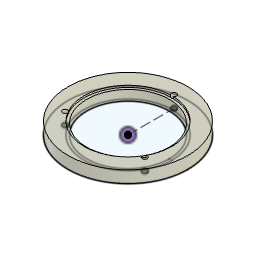
Kattolampun adapteri v5 (Autodesk Fusion 360 design; units mm, degrees)
Autodesk Fusion 360 part; units mm, degrees
sketch "Base" plane through (0, 0, 0) normal (0, 0, 1) x (1, 0, 0)
  circle A0 centre (0, 0) radius 45
  circle A1 centre (0, 0) radius 47.75
  circle A2 centre (0, 0) radius 65
  line L0 (0, 0) -> (0, 50) construction
  circle A3 centre (0, 50) radius 2.75
  circle A4 centre (-43.3013, -25) radius 2.75
  circle A5 centre (43.3013, -25) radius 2.75
  dimension "d6" = 90
  dimension "d7" = 95.5
  dimension "d8" = 130
  dimension "d12" = 50
  dimension "d13" = 5.5
  dimension "d15" = 360
  constraint coincident A0.centre A1.centre
  constraint vertical L0
  constraint coincident L0.end A3.centre
  measures "d6" diameter of A0
  measures "d7" diameter of A1
  measures "d8" diameter of A2
  measures "d12" distance of A0.centre L0.end
  measures "d13" diameter of A3
extrude "Extrude1" add sketch "Base" along normal blind 13 contours A0 | A1 A3 A4 A5 | A2
extrude "Extrude2" add sketch "Base" along normal up to surface (11 mm away) from surface at 2 contours A1 A3 A4 A5 | A1 A3 | A1 A5 | A1 A4 picked at (0, 47.5815) picked at (41.2068, -23.7907) picked at (-41.224, -23.7621)
extrude "Extrude3" add sketch "Base" along normal up to surface (5 mm away) from surface at 8 contours A1 A3 | A1 A3 | A1 A5 | A1 A5 | A1 A4 | A1 A4
extrude "Extrude4" cut sketch "Base" along normal up to surface (13 mm away) contours A1 A3 | A1 A5 | A1 A4 picked at (-0.0423, 49.4138) picked at (42.7651, -24.7549) picked at (-42.7945, -24.7074)
extrude "Extrude5" cut sketch "Base" along normal up to surface (13 mm away) contours A0
extrude "Extrude6" cut sketch "Base" along normal up to surface (13 mm away) contours A1 A3 | A1 A3 | A1 A5 | A1 A5 | A1 A4 | A1 A4
extrude "Extrude7" cut sketch "Base" against normal blind 2 from surface at 13 contours A1 A3 A4 A5
equation "adapterInnerHoleDiameter = 89 mm" comment "Valkoisen välipalikan pienempi hole"
equation "adapterFlangeDepth = 2 mm" comment "Valkoisen välipalikan huulloksen syvyys"
equation "adapterFlangeDiameter = 94.5 mm" comment "Valkoisen välipalikan huulloksen halkaisija"
equation "plafondBaseDiameter = 130 mm" comment "Plafondilampun pohjan halkaisija"
equation "plafondBaseScrewDistance = 87 mm" comment "Plafondin kiinnitysruuvien etäisyys"
equation "d6 = adapterInnerHoleDiameter + shrinkageTolerance"
equation "d7 = adapterFlangeDiameter + shrinkageTolerance"
equation "d8 = plafondBaseDiameter"
equation "adapterInnerHoleDepth = 11 mm" comment "Valkoisen välipalikan syvyys"
equation "heatInsertDiameter = 5.5 mm" comment "M4 brass heat insert"
equation "heatInsertLength = 8 mm" comment "M4 brass heat insert"
equation "d12 = adapterFlangeDiameter / 2 + heatInsertDiameter / 2"
equation "d13 = heatInsertDiameter"
equation "d16 = adapterFlangeDepth + adapterInnerHoleDepth"
equation "d18 = adapterFlangeDepth"
equation "d21 = heatInsertLength"
equation "shrinkageTolerance = 1 mm" comment "Account printing material shrinkage"
equation "d32 = -adapterFlangeDepth"
named bodies: "Adapter"
